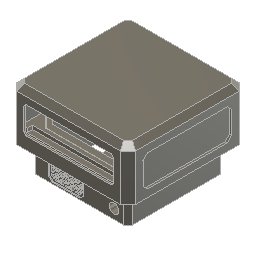
body (Autodesk Fusion 360 design; units mm, degrees)
part number: 2025-12-12-12-39-30-884
part number: 2025-12-12-12-40-35-354
part number: 2025-12-12-12-40-41-238
part number: 2025-12-13-11-33-40-663
Autodesk Fusion 360 part; units mm, degrees
(part 1 of 2)
sketch "Sketch1" plane through (0, 0, 0) normal (0, 1, 0) x (1, 0, 0) in component "Bottom"
  line L0 (-45, 45) -> (45, 45)
  line L1 (45, 45) -> (45, -45)
  line L2 (45, -45) -> (-45, -45)
  line L3 (-45, -45) -> (-45, 45)
  line L4 (-45, 45) -> (45, -45) construction
  line L5 (45, 45) -> (-45, -45) construction
  line L6 (37, -37) -> (-37, -37)
  line L7 (-37, -37) -> (-37, 37)
  line L8 (-37, 37) -> (37, 37)
  line L9 (37, 37) -> (37, -37)
  dimension "d1" = 90
  dimension "d2" = 90
  dimension "d3" = 8
  constraint horizontal L0
  constraint perpendicular L0 L1
  constraint parallel L0 L2
  constraint parallel L1 L3
  constraint coincident L4 origin
  constraint coincident L5 origin
  measures "d1" distance of L1.end L2.end
  measures "d2" distance of L0.end L1.end
extrude "Extrude1" add sketch "Sketch1" along normal blind 40 makes body 1 in component "Bottom"
sketch "Sketch2" plane through (0, 0, 0) normal (0, 0, 1) x (1, 0, 0) in component "Bottom"
ref_plane "WorkPlane1" through (0, 25, 0) normal (0, 1, 0) x (0, 0, 1) in component "Top"
sketch "Sketch1 (2)" plane through (0, 25, 0) normal (0, 1, 0) x (1, 0, 0) in component "Top"
  line L0 (55, 55) -> (-55, 55)
  line L1 (-55, 55) -> (-55, -55)
  line L2 (-55, -55) -> (55, -55)
  line L3 (55, -55) -> (55, 55)
  line L4 (55, 55) -> (-55, -55) construction
  line L5 (-55, 55) -> (55, -55) construction
  dimension "d7" = 110
  dimension "d8" = 110
  constraint horizontal L0
  constraint perpendicular L0 L1
  constraint parallel L0 L2
  constraint parallel L1 L3
  constraint coincident L4 origin
  constraint coincident L5 origin
  measures "d7" distance of L1.end L2.end
  measures "d8" distance of L0.end L1.end
extrude "Extrude1'" add sketch "Sketch1 (2)" along normal blind 48 separate body makes body 2 in component "Top"
shell "Shell1" thickness 8 removed faces 1 at (-18.3333, 25, -18.3333) on bodies 2 in component "Top"
sketch "Sketch2 (2)" plane through (0, 25, 0) normal (0, -1, 0) x (1, 0, 0) in component "Top"
  line L0 (-47, 47) -> (47, 47)
  line L1 (47, 47) -> (47, -47)
  line L2 (47, -47) -> (-47, -47)
  line L3 (-47, -47) -> (-47, 47)
  line L4 (55, -55) -> (55, 55)
  line L5 (55, 55) -> (-55, 55)
  line L6 (-55, 55) -> (-55, -55)
  line L7 (-55, -55) -> (55, -55)
  line L8 (51, -51) -> (-51, -51)
  line L9 (-51, -51) -> (-51, 51)
  line L10 (-51, 51) -> (51, 51)
  line L11 (51, 51) -> (51, -51)
  dimension "d12" = -4
extrude "Extrude2" cut sketch "Sketch2 (2)" against normal blind 10 contours L8 L9 L10 L11 bodies 2 in component "Top"
sketch "Sketch3" plane through (0, 0, 55) normal (0, 0, 1) x (1, 0, 0) in component "Top"
  line L0 (-55, 25) -> (55, 25)
  line L1 (55, 25) -> (55, 73)
  line L2 (55, 73) -> (-55, 73)
  line L3 (-55, 73) -> (-55, 25)
  line L4 (0, 73) -> (0, 25) construction
  line L5 (-41.5, 61.5) -> (41.5, 61.5)
  line L6 (41.5, 61.5) -> (41.5, 36.5)
  line L7 (41.5, 36.5) -> (-41.5, 36.5)
  line L8 (-41.5, 36.5) -> (-41.5, 61.5)
  line L9 (-41.5, 61.5) -> (41.5, 36.5) construction
  line L10 (41.5, 61.5) -> (-41.5, 36.5) construction
  line L11 (50.5, 66) -> (-50.5, 66)
  line L12 (-50.5, 66) -> (-50.5, 32)
  line L13 (-50.5, 32) -> (50.5, 32)
  line L14 (50.5, 32) -> (50.5, 66)
  line L15 (50.5, 66) -> (-50.5, 32) construction
  line L16 (-50.5, 66) -> (50.5, 32) construction
  point P0 (0, 49)
  point P1 (0, 49)
  dimension "d15" = 83
  dimension "d16" = 25
  dimension "d29" = 101
  dimension "d30" = 34
  constraint midpoint L2 L4.start
  constraint midpoint L0 L4.end
  constraint horizontal L5
  constraint perpendicular L5 L6
  constraint parallel L5 L7
  constraint parallel L6 L8
  constraint coincident L9 P1
  constraint coincident L10 P1
  constraint midpoint L4 P1
  constraint horizontal L11
  constraint perpendicular L11 L12
  constraint parallel L11 L13
  constraint parallel L12 L14
  constraint coincident L15 P1
  constraint coincident L16 P1
  constraint coincident P1 P0
  measures "d15" distance of L6.end L7.end
  measures "d16" distance of L5.end L6.end
  measures "d29" distance of L12.end L13.end
  measures "d30" distance of L11.end L12.end
extrude "Extrude3" cut sketch "Sketch3" against normal blind 8 contours L5 L6 L7 L8 bodies 2 in component "Top"
sketch "Sketch3 (2)" plane through (0, 0, 45) normal (0, 0, 1) x (1, 0, 0) in component "Bottom"
  line L0 (-45, 0) -> (45, 0)
  line L1 (45, 0) -> (45, 40)
  line L2 (45, 40) -> (-45, 40)
  line L3 (-45, 40) -> (-45, 0)
sketch "Sketch4" plane through (0, 40, 0) normal (0, 1, 0) x (-1, 0, 0) in component "Bottom"
  line L0 (37, -37) -> (-37, -37)
  line L1 (-37, -37) -> (-37, 37)
  line L2 (-37, 37) -> (37, 37)
  line L3 (37, 37) -> (37, -37)
  line L4 (45, 45) -> (-45, 45)
  line L5 (-45, 45) -> (-45, -45)
  line L6 (-45, -45) -> (45, -45)
  line L7 (45, -45) -> (45, 45)
  line L8 (43, 43) -> (-43, 43)
  line L9 (-43, 43) -> (-43, -43)
  line L10 (-43, -43) -> (43, -43)
  line L11 (43, -43) -> (43, 43)
  dimension "d20" = -2
extrude "Extrude2'" cut sketch "Sketch4" against normal blind 12 contours L4 L5 L6 L7 bodies 1 in component "Bottom"
sketch "Sketch4 (2)" plane through (0, 35, 0) normal (0, -1, 0) x (1, 0, 0) in component "Top"
  line L0 (47, -47) -> (-47, -47)
  line L1 (-47, -47) -> (-47, 47)
  line L2 (-47, 47) -> (47, 47)
  line L3 (47, 47) -> (47, -47)
  line L4 (51, 51) -> (-51, 51)
  line L5 (-51, 51) -> (-51, -51)
  line L6 (-51, -51) -> (51, -51)
  line L7 (51, -51) -> (51, 51)
  line L8 (43, -43) -> (-43, -43)
  line L9 (-43, -43) -> (-43, 43)
  line L10 (-43, 43) -> (43, 43)
  line L11 (43, 43) -> (43, -43)
  line L12 (-37, -37) -> (37, -37)
  line L13 (37, -37) -> (37, 37)
  line L14 (37, 37) -> (-37, 37)
  line L15 (-37, 37) -> (-37, -37)
extrude "Extrude4" add sketch "Sketch4 (2)" against normal blind 5 contours L0 L1 L2 L3 bodies 2 in component "Top"
sketch "Sketch5" plane through (0, 40, 0) normal (0, 1, 0) x (-1, 0, 0) in component "Top"
  line L0 (-43, 43) -> (43, 43)
  line L1 (43, 43) -> (43, -43)
  line L2 (43, -43) -> (-43, -43)
  line L3 (-43, -43) -> (-43, 43)
  line L4 (47, 47) -> (41.5, 47)
  line L5 (-47, 47) -> (-47, -47)
  line L6 (-47, -47) -> (47, -47)
  line L7 (47, -47) -> (47, 47)
  line L8 (43, -33) -> (33, -43)
  line L9 (43, -33) -> (43, -43)
  line L10 (43, -43) -> (33, -43)
  line L11 (-43, -43) -> (-33, -43)
  line L12 (-33, -43) -> (-43, -33)
  line L13 (-43, -43) -> (-43, -33)
  line L14 (-43, 43) -> (-43, 33)
  line L15 (-43, 33) -> (-33, 43)
  line L16 (-33, 43) -> (-43, 43)
  line L17 (43, 43) -> (43, 33)
  line L18 (43, 33) -> (33, 43)
  line L19 (33, 43) -> (43, 43)
  line L20 (41.5, 47) -> (-41.5, 47)
  line L21 (-41.5, 47) -> (-47, 47)
  dimension "d25" = 10
  constraint coincident L1 L8.start
  constraint coincident L2 L8.end
  constraint coincident L1.end L2.start
  constraint coincident L2.end L3.start
  constraint coincident L2 L11.end
  constraint coincident L3 L12.end
  constraint coincident L0.start L3.end
  constraint coincident L3 L14.end
  constraint coincident L0 L15.end
  constraint coincident L0.end L1.start
  constraint coincident L1 L17.end
  constraint coincident L0 L18.end
  constraint equal L9 L10
  constraint equal L10 L11
  constraint equal L11 L13
  constraint equal L17 L19
  constraint equal L10 L17
  constraint equal L14 L16
  constraint equal L10 L14
  measures "d25" distance of L8.end L1.end
extrude "Extrude5" add sketch "Sketch5" against normal blind 2 contours L0 L3 L14 L15 L16 | L0 L1 L17 L18 L19 | L2 L3 L11 L12 L13 | L1 L2 L8 L9 L10 bodies 2 in component "Top"
combine "Combine1" operation cut target body 1 tool bodies 2 keep tools in component "Bottom"
move_face "OffsetFaces1" offset -0.2 8 faces at (-43, 36, -11) (11, 36, -43) (-39.6667, 39.3333, -36.3333) (43, 36, 11) (36.3333, 39.3333, -39.6667) (-11, 36, 43) (39.6667, 39.3333, 36.3333) (-39.6667, 39.3333, 36.3333) on bodies 2 in component "Top"
extrude "Extrude6" cut 1 faces at (-45.1667, 55.5, 47) along direction (0, 0, 1) blind 6.5 on bodies 2 bodies 2 in component "Top"
sketch "Sketch6" plane through (0, 40, 0) normal (0, 1, 0) x (-1, 0, 0) in component "Top"
  line L0 (-33.0828, 43.2) -> (33.0828, 43.2)
  line L1 (33.0828, 43.2) -> (43.2, 33.0828)
  line L2 (43.2, 33.0828) -> (43.2, -33.0828)
  line L3 (43.2, -33.0828) -> (33.0828, -43.2)
  line L4 (33.0828, -43.2) -> (-33.0828, -43.2)
  line L5 (-33.0828, -43.2) -> (-43.2, -33.0828)
  line L6 (-43.2, -33.0828) -> (-43.2, 33.0828)
  line L7 (-43.2, 33.0828) -> (-33.0828, 43.2)
  line L8 (41.5, 47) -> (-41.5, 47)
  line L9 (-41.5, 47) -> (-41.5, 53.5)
  line L10 (-41.5, 53.5) -> (-47, 53.5)
  line L11 (-47, 53.5) -> (-47, -47)
  line L12 (-47, -47) -> (47, -47)
  line L13 (47, -47) -> (47, 53.5)
  line L14 (47, 53.5) -> (41.5, 53.5)
  line L15 (41.5, 53.5) -> (41.5, 47)
  line L16 (47, 53.5) -> (-47, 53.5)
  line L17 (-47, 53.5) -> (-47, 52)
  line L18 (-47, 52) -> (47, 52)
  line L19 (47, 52) -> (47, 53.5)
  dimension "d33" = 1.5
  constraint horizontal L16
  constraint vertical L17
  constraint horizontal L18
  constraint vertical L19
  constraint coincident L11 L17.end
  constraint coincident L13.end L14.start
  measures "d33" distance of L13.end L18.end
extrude "Extrude7" cut sketch "Sketch6" against normal blind 5 contours L9 L15 L16 L18 | L13 L14 L15 L16 L18 L19 | L9 L10 L11 L16 L17 L18 bodies 2 in component "Top"
chamfer "Chamfer1" distance 7 angle 45 4 edges at (-55, 49, 55) (55, 49, 55) (55, 49, -55) (-55, 49, -55) on bodies 2 in component "Top"
chamfer "Chamfer2" distance 5 angle 45 4 edges at (51, 30, 51) (-51, 30, 51) (51, 30, -51) (-51, 30, -51) on bodies 2 in component "Top"
chamfer "Chamfer3" distance 4 angle 45 2 edges at (-47, 52.5, -47) (47, 52.5, -47) on bodies 2 in component "Top"
chamfer "Chamfer4" distance 5 angle 45 8 edges at (-55, 73, 0) (-51.5, 73, 51.5) (0, 73, 55) (51.5, 73, 51.5) (55, 73, 0) (0, 73, -55) (51.5, 73, -51.5) (-51.5, 73, -51.5) on bodies 2 in component "Top"
chamfer "Chamfer1'" distance 4 angle 45 12 edges at (-45, 14, -45) (-45, 14, 45) (45, 14, -45) (-43, 33, -43) (-43, 33, 43) (45, 14, 45) (43, 33, 43) (43, 33, -43) (-37, 20, 37) (37, 20, 37) (37, 20, -37) (-37, 20, -37) on bodies 1 in component "Bottom"
sketch "Sketch5 (2)" plane through (0, 0, 37) normal (0, 0, -1) x (-1, 0, 0) in component "Bottom"
  line L0 (-33, 40) -> (-33, 0)
  line L1 (-33, 0) -> (33, 0)
  line L2 (33, 0) -> (33, 40)
  line L3 (33, 40) -> (-33, 40)
  line L4 (-2, 23) -> (27, 23)
  line L5 (27, 23) -> (27, 3)
  line L6 (27, 3) -> (-2, 3)
  line L7 (-2, 3) -> (-2, 23)
  line L8 (-2, 23) -> (27, 3) construction
  line L9 (27, 23) -> (-2, 3) construction
  line L10 (-5.5, 25.5) -> (30.5, 25.5)
  line L11 (30.5, 25.5) -> (30.5, 0.5)
  line L12 (30.5, 0.5) -> (-5.5, 0.5)
  line L13 (-5.5, 0.5) -> (-5.5, 25.5)
  line L14 (-5.5, 25.5) -> (30.5, 0.5) construction
  line L15 (30.5, 25.5) -> (-5.5, 0.5) construction
  point P0 (12.5, 13)
  point P1 (12.5, 13)
  dimension "d41" = 29
  dimension "d42" = 3
  dimension "d43" = 6
  dimension "d46" = 36
  dimension "d47" = 25
  constraint horizontal L4
  constraint perpendicular L4 L5
  constraint parallel L4 L6
  constraint parallel L5 L7
  constraint coincident L8 P1
  constraint coincident L9 P1
  constraint horizontal L10
  constraint perpendicular L10 L11
  constraint parallel L10 L12
  constraint parallel L11 L13
  constraint coincident L14 P1
  constraint coincident L15 P1
  constraint coincident P1 P0
  measures "d41" distance of L5.end L6.end
  measures "d42" distance of L1 L6
  measures "d43" distance of L2 L5
  measures "d46" distance of L11.end L12.end
  measures "d47" distance of L10.end L11.end
sketch "Sketch6 (2)" plane through (0, 0, 45) normal (0, 0, 1) x (1, 0, 0) in component "Bottom"
  line L0 (2, 23) -> (-27, 23)
  line L1 (2, 3) -> (2, 23)
  line L2 (-27, 23) -> (-27, 3)
  line L3 (-27, 3) -> (2, 3)
  line L4 (-13.6547, 15) -> (-14.8094, 13)
  line L5 (-14.8094, 13) -> (-13.6547, 11)
  line L6 (-13.6547, 11) -> (-11.3453, 11)
  line L7 (-11.3453, 11) -> (-10.1906, 13)
  line L8 (-10.1906, 13) -> (-11.3453, 15)
  line L9 (-11.3453, 15) -> (-13.6547, 15)
  line L10 (-11.3453, 15) -> (-10.0463, 15.75)
  line L11 (2.5111, 39) -> (0.2017, 39)
  line L12 (0.2017, 39) -> (-0.953, 37)
  line L13 (-0.953, 37) -> (0.2017, 35)
  line L14 (0.2017, 35) -> (2.5111, 35)
  line L15 (2.5111, 35) -> (3.6658, 37)
  line L16 (3.6658, 37) -> (2.5111, 39)
  line L17 (-2.1077, 36.3333) -> (-4.4171, 36.3333)
  line L18 (-4.4171, 36.3333) -> (-5.5718, 34.3333)
  line L19 (-5.5718, 34.3333) -> (-4.4171, 32.3333)
  line L20 (-4.4171, 32.3333) -> (-2.1077, 32.3333)
  line L21 (-2.1077, 32.3333) -> (-0.953, 34.3333)
  line L22 (-0.953, 34.3333) -> (-2.1077, 36.3333)
  line L23 (-6.7265, 33.6667) -> (-9.0359, 33.6667)
  line L24 (-9.0359, 33.6667) -> (-10.1906, 31.6667)
  line L25 (-10.1906, 31.6667) -> (-9.0359, 29.6667)
  line L26 (-9.0359, 29.6667) -> (-6.7265, 29.6667)
  line L27 (-6.7265, 29.6667) -> (-5.5718, 31.6667)
  line L28 (-5.5718, 31.6667) -> (-6.7265, 33.6667)
  line L29 (-11.3453, 31) -> (-13.6547, 31)
  line L30 (-13.6547, 31) -> (-14.8094, 29)
  line L31 (-14.8094, 29) -> (-13.6547, 27)
  line L32 (-13.6547, 27) -> (-11.3453, 27)
  line L33 (-11.3453, 27) -> (-10.1906, 29)
  line L34 (-10.1906, 29) -> (-11.3453, 31)
  line L35 (-15.9641, 28.3333) -> (-18.2735, 28.3333)
  line L36 (-18.2735, 28.3333) -> (-19.4282, 26.3333)
  line L37 (-19.4282, 26.3333) -> (-18.2735, 24.3333)
  line L38 (-18.2735, 24.3333) -> (-15.9641, 24.3333)
  line L39 (-15.9641, 24.3333) -> (-14.8094, 26.3333)
  line L40 (-14.8094, 26.3333) -> (-15.9641, 28.3333)
  line L41 (-20.5829, 25.6667) -> (-22.8923, 25.6667)
  line L42 (-22.8923, 25.6667) -> (-24.047, 23.6667)
  line L43 (-24.047, 23.6667) -> (-22.8923, 21.6667)
  line L44 (-22.8923, 21.6667) -> (-20.5829, 21.6667)
  line L45 (-20.5829, 21.6667) -> (-19.4282, 23.6667)
  line L46 (-19.4282, 23.6667) -> (-20.5829, 25.6667)
  line L47 (-25.2017, 23) -> (-27.5111, 23)
  line L48 (-27.5111, 23) -> (-28.6658, 21)
  line L49 (-28.6658, 21) -> (-27.5111, 19)
  line L50 (-27.5111, 19) -> (-25.2017, 19)
  line L51 (-25.2017, 19) -> (-24.047, 21)
  line L52 (-24.047, 21) -> (-25.2017, 23)
  line L53 (2.5111, 33.6667) -> (0.2017, 33.6667)
  line L54 (0.2017, 33.6667) -> (-0.953, 31.6667)
  line L55 (-0.953, 31.6667) -> (0.2017, 29.6667)
  line L56 (0.2017, 29.6667) -> (2.5111, 29.6667)
  line L57 (2.5111, 29.6667) -> (3.6658, 31.6667)
  line L58 (3.6658, 31.6667) -> (2.5111, 33.6667)
  line L59 (-2.1077, 31) -> (-4.4171, 31)
  line L60 (-4.4171, 31) -> (-5.5718, 29)
  line L61 (-5.5718, 29) -> (-4.4171, 27)
  line L62 (-4.4171, 27) -> (-2.1077, 27)
  line L63 (-2.1077, 27) -> (-0.953, 29)
  line L64 (-0.953, 29) -> (-2.1077, 31)
  line L65 (-6.7265, 28.3333) -> (-9.0359, 28.3333)
  line L66 (-9.0359, 28.3333) -> (-10.1906, 26.3333)
  line L67 (-10.1906, 26.3333) -> (-9.0359, 24.3333)
  line L68 (-9.0359, 24.3333) -> (-6.7265, 24.3333)
  line L69 (-6.7265, 24.3333) -> (-5.5718, 26.3333)
  line L70 (-5.5718, 26.3333) -> (-6.7265, 28.3333)
  line L71 (-11.3453, 25.6667) -> (-13.6547, 25.6667)
  line L72 (-13.6547, 25.6667) -> (-14.8094, 23.6667)
  line L73 (-14.8094, 23.6667) -> (-13.6547, 21.6667)
  line L74 (-13.6547, 21.6667) -> (-11.3453, 21.6667)
  line L75 (-11.3453, 21.6667) -> (-10.1906, 23.6667)
  line L76 (-10.1906, 23.6667) -> (-11.3453, 25.6667)
  line L77 (-15.9641, 23) -> (-18.2735, 23)
  line L78 (-18.2735, 23) -> (-19.4282, 21)
  line L79 (-19.4282, 21) -> (-18.2735, 19)
  line L80 (-18.2735, 19) -> (-15.9641, 19)
  line L81 (-15.9641, 19) -> (-14.8094, 21)
  line L82 (-14.8094, 21) -> (-15.9641, 23)
  line L83 (-20.5829, 20.3333) -> (-22.8923, 20.3333)
  line L84 (-22.8923, 20.3333) -> (-24.047, 18.3333)
  line L85 (-24.047, 18.3333) -> (-22.8923, 16.3333)
  line L86 (-22.8923, 16.3333) -> (-20.5829, 16.3333)
  line L87 (-20.5829, 16.3333) -> (-19.4282, 18.3333)
  line L88 (-19.4282, 18.3333) -> (-20.5829, 20.3333)
  line L89 (-25.2017, 17.6667) -> (-27.5111, 17.6667)
  line L90 (-27.5111, 17.6667) -> (-28.6658, 15.6667)
  line L91 (-28.6658, 15.6667) -> (-27.5111, 13.6667)
  line L92 (-27.5111, 13.6667) -> (-25.2017, 13.6667)
  line L93 (-25.2017, 13.6667) -> (-24.047, 15.6667)
  line L94 (-24.047, 15.6667) -> (-25.2017, 17.6667)
  line L95 (2.5111, 28.3333) -> (0.2017, 28.3333)
  line L96 (0.2017, 28.3333) -> (-0.953, 26.3333)
  line L97 (-0.953, 26.3333) -> (0.2017, 24.3333)
  line L98 (0.2017, 24.3333) -> (2.5111, 24.3333)
  line L99 (2.5111, 24.3333) -> (3.6658, 26.3333)
  line L100 (3.6658, 26.3333) -> (2.5111, 28.3333)
  line L101 (-2.1077, 25.6667) -> (-4.4171, 25.6667)
  line L102 (-4.4171, 25.6667) -> (-5.5718, 23.6667)
  line L103 (-5.5718, 23.6667) -> (-4.4171, 21.6667)
  line L104 (-4.4171, 21.6667) -> (-2.1077, 21.6667)
  line L105 (-2.1077, 21.6667) -> (-0.953, 23.6667)
  line L106 (-0.953, 23.6667) -> (-2.1077, 25.6667)
  line L107 (-6.7265, 23) -> (-9.0359, 23)
  line L108 (-9.0359, 23) -> (-10.1906, 21)
  line L109 (-10.1906, 21) -> (-9.0359, 19)
  line L110 (-9.0359, 19) -> (-6.7265, 19)
  line L111 (-6.7265, 19) -> (-5.5718, 21)
  line L112 (-5.5718, 21) -> (-6.7265, 23)
  line L113 (-11.3453, 20.3333) -> (-13.6547, 20.3333)
  line L114 (-13.6547, 20.3333) -> (-14.8094, 18.3333)
  line L115 (-14.8094, 18.3333) -> (-13.6547, 16.3333)
  line L116 (-13.6547, 16.3333) -> (-11.3453, 16.3333)
  line L117 (-11.3453, 16.3333) -> (-10.1906, 18.3333)
  line L118 (-10.1906, 18.3333) -> (-11.3453, 20.3333)
  line L119 (-15.9641, 17.6667) -> (-18.2735, 17.6667)
  line L120 (-18.2735, 17.6667) -> (-19.4282, 15.6667)
  line L121 (-19.4282, 15.6667) -> (-18.2735, 13.6667)
  line L122 (-18.2735, 13.6667) -> (-15.9641, 13.6667)
  line L123 (-15.9641, 13.6667) -> (-14.8094, 15.6667)
  line L124 (-14.8094, 15.6667) -> (-15.9641, 17.6667)
  line L125 (-20.5829, 15) -> (-22.8923, 15)
  line L126 (-22.8923, 15) -> (-24.047, 13)
  line L127 (-24.047, 13) -> (-22.8923, 11)
  line L128 (-22.8923, 11) -> (-20.5829, 11)
  line L129 (-20.5829, 11) -> (-19.4282, 13)
  line L130 (-19.4282, 13) -> (-20.5829, 15)
  line L131 (-25.2017, 12.3333) -> (-27.5111, 12.3333)
  line L132 (-27.5111, 12.3333) -> (-28.6658, 10.3333)
  line L133 (-28.6658, 10.3333) -> (-27.5111, 8.3333)
  line L134 (-27.5111, 8.3333) -> (-25.2017, 8.3333)
  line L135 (-25.2017, 8.3333) -> (-24.047, 10.3333)
  line L136 (-24.047, 10.3333) -> (-25.2017, 12.3333)
  line L137 (2.5111, 23) -> (0.2017, 23)
  line L138 (0.2017, 23) -> (-0.953, 21)
  line L139 (-0.953, 21) -> (0.2017, 19)
  line L140 (0.2017, 19) -> (2.5111, 19)
  line L141 (2.5111, 19) -> (3.6658, 21)
  line L142 (3.6658, 21) -> (2.5111, 23)
  line L143 (-2.1077, 20.3333) -> (-4.4171, 20.3333)
  line L144 (-4.4171, 20.3333) -> (-5.5718, 18.3333)
  line L145 (-5.5718, 18.3333) -> (-4.4171, 16.3333)
  line L146 (-4.4171, 16.3333) -> (-2.1077, 16.3333)
  line L147 (-2.1077, 16.3333) -> (-0.953, 18.3333)
  line L148 (-0.953, 18.3333) -> (-2.1077, 20.3333)
  line L149 (-6.7265, 17.6667) -> (-9.0359, 17.6667)
  line L150 (-9.0359, 17.6667) -> (-10.1906, 15.6667)
  line L151 (-10.1906, 15.6667) -> (-9.0359, 13.6667)
  line L152 (-9.0359, 13.6667) -> (-6.7265, 13.6667)
  line L153 (-6.7265, 13.6667) -> (-5.5718, 15.6667)
  line L154 (-5.5718, 15.6667) -> (-6.7265, 17.6667)
  line L155 (-15.9641, 12.3333) -> (-18.2735, 12.3333)
  line L156 (-18.2735, 12.3333) -> (-19.4282, 10.3333)
  line L157 (-19.4282, 10.3333) -> (-18.2735, 8.3333)
  line L158 (-18.2735, 8.3333) -> (-15.9641, 8.3333)
  line L159 (-15.9641, 8.3333) -> (-14.8094, 10.3333)
  line L160 (-14.8094, 10.3333) -> (-15.9641, 12.3333)
  line L161 (-20.5829, 9.6667) -> (-22.8923, 9.6667)
  line L162 (-22.8923, 9.6667) -> (-24.047, 7.6667)
  line L163 (-24.047, 7.6667) -> (-22.8923, 5.6667)
  line L164 (-22.8923, 5.6667) -> (-20.5829, 5.6667)
  line L165 (-20.5829, 5.6667) -> (-19.4282, 7.6667)
  line L166 (-19.4282, 7.6667) -> (-20.5829, 9.6667)
  line L167 (-25.2017, 7) -> (-27.5111, 7)
  line L168 (-27.5111, 7) -> (-28.6658, 5)
  line L169 (-28.6658, 5) -> (-27.5111, 3)
  line L170 (-27.5111, 3) -> (-25.2017, 3)
  line L171 (-25.2017, 3) -> (-24.047, 5)
  line L172 (-24.047, 5) -> (-25.2017, 7)
  line L173 (2.5111, 17.6667) -> (0.2017, 17.6667)
  line L174 (0.2017, 17.6667) -> (-0.953, 15.6667)
  line L175 (-0.953, 15.6667) -> (0.2017, 13.6667)
  line L176 (0.2017, 13.6667) -> (2.5111, 13.6667)
  line L177 (2.5111, 13.6667) -> (3.6658, 15.6667)
  line L178 (3.6658, 15.6667) -> (2.5111, 17.6667)
  line L179 (-2.1077, 15) -> (-4.4171, 15)
  line L180 (-4.4171, 15) -> (-5.5718, 13)
  line L181 (-5.5718, 13) -> (-4.4171, 11)
  line L182 (-4.4171, 11) -> (-2.1077, 11)
  line L183 (-2.1077, 11) -> (-0.953, 13)
  line L184 (-0.953, 13) -> (-2.1077, 15)
  line L185 (-6.7265, 12.3333) -> (-9.0359, 12.3333)
  line L186 (-9.0359, 12.3333) -> (-10.1906, 10.3333)
  line L187 (-10.1906, 10.3333) -> (-9.0359, 8.3333)
  line L188 (-9.0359, 8.3333) -> (-6.7265, 8.3333)
  line L189 (-6.7265, 8.3333) -> (-5.5718, 10.3333)
  line L190 (-5.5718, 10.3333) -> (-6.7265, 12.3333)
  line L191 (-11.3453, 9.6667) -> (-13.6547, 9.6667)
  line L192 (-13.6547, 9.6667) -> (-14.8094, 7.6667)
  line L193 (-14.8094, 7.6667) -> (-13.6547, 5.6667)
  line L194 (-13.6547, 5.6667) -> (-11.3453, 5.6667)
  line L195 (-11.3453, 5.6667) -> (-10.1906, 7.6667)
  line L196 (-10.1906, 7.6667) -> (-11.3453, 9.6667)
  line L197 (-15.9641, 7) -> (-18.2735, 7)
  line L198 (-18.2735, 7) -> (-19.4282, 5)
  line L199 (-19.4282, 5) -> (-18.2735, 3)
  line L200 (-18.2735, 3) -> (-15.9641, 3)
  line L201 (-15.9641, 3) -> (-14.8094, 5)
  line L202 (-14.8094, 5) -> (-15.9641, 7)
  line L203 (-20.5829, 4.3333) -> (-22.8923, 4.3333)
  line L204 (-22.8923, 4.3333) -> (-24.047, 2.3333)
  line L205 (-24.047, 2.3333) -> (-22.8923, 0.3333)
  line L206 (-22.8923, 0.3333) -> (-20.5829, 0.3333)
  line L207 (-20.5829, 0.3333) -> (-19.4282, 2.3333)
  line L208 (-19.4282, 2.3333) -> (-20.5829, 4.3333)
  line L209 (-25.2017, 1.6667) -> (-27.5111, 1.6667)
  line L210 (-27.5111, 1.6667) -> (-28.6658, -0.3333)
  line L211 (-28.6658, -0.3333) -> (-27.5111, -2.3333)
  line L212 (-27.5111, -2.3333) -> (-25.2017, -2.3333)
  line L213 (-25.2017, -2.3333) -> (-24.047, -0.3333)
  line L214 (-24.047, -0.3333) -> (-25.2017, 1.6667)
  line L215 (2.5111, 12.3333) -> (0.2017, 12.3333)
  line L216 (0.2017, 12.3333) -> (-0.953, 10.3333)
  line L217 (-0.953, 10.3333) -> (0.2017, 8.3333)
  line L218 (0.2017, 8.3333) -> (2.5111, 8.3333)
  line L219 (2.5111, 8.3333) -> (3.6658, 10.3333)
  line L220 (3.6658, 10.3333) -> (2.5111, 12.3333)
  line L221 (-2.1077, 9.6667) -> (-4.4171, 9.6667)
  line L222 (-4.4171, 9.6667) -> (-5.5718, 7.6667)
  line L223 (-5.5718, 7.6667) -> (-4.4171, 5.6667)
  line L224 (-4.4171, 5.6667) -> (-2.1077, 5.6667)
  line L225 (-2.1077, 5.6667) -> (-0.953, 7.6667)
  line L226 (-0.953, 7.6667) -> (-2.1077, 9.6667)
  line L227 (-6.7265, 7) -> (-9.0359, 7)
  line L228 (-9.0359, 7) -> (-10.1906, 5)
  line L229 (-10.1906, 5) -> (-9.0359, 3)
  line L230 (-9.0359, 3) -> (-6.7265, 3)
  line L231 (-6.7265, 3) -> (-5.5718, 5)
  line L232 (-5.5718, 5) -> (-6.7265, 7)
  line L233 (-11.3453, 4.3333) -> (-13.6547, 4.3333)
  line L234 (-13.6547, 4.3333) -> (-14.8094, 2.3333)
  line L235 (-14.8094, 2.3333) -> (-13.6547, 0.3333)
  line L236 (-13.6547, 0.3333) -> (-11.3453, 0.3333)
  line L237 (-11.3453, 0.3333) -> (-10.1906, 2.3333)
  line L238 (-10.1906, 2.3333) -> (-11.3453, 4.3333)
  line L239 (-15.9641, 1.6667) -> (-18.2735, 1.6667)
  line L240 (-18.2735, 1.6667) -> (-19.4282, -0.3333)
  line L241 (-19.4282, -0.3333) -> (-18.2735, -2.3333)
  line L242 (-18.2735, -2.3333) -> (-15.9641, -2.3333)
  line L243 (-15.9641, -2.3333) -> (-14.8094, -0.3333)
  line L244 (-14.8094, -0.3333) -> (-15.9641, 1.6667)
  line L245 (-20.5829, -1) -> (-22.8923, -1)
  line L246 (-22.8923, -1) -> (-24.047, -3)
  line L247 (-24.047, -3) -> (-22.8923, -5)
  line L248 (-22.8923, -5) -> (-20.5829, -5)
  line L249 (-20.5829, -5) -> (-19.4282, -3)
  line L250 (-19.4282, -3) -> (-20.5829, -1)
  line L251 (-25.2017, -3.6667) -> (-27.5111, -3.6667)
  line L252 (-27.5111, -3.6667) -> (-28.6658, -5.6667)
  line L253 (-28.6658, -5.6667) -> (-27.5111, -7.6667)
  line L254 (-27.5111, -7.6667) -> (-25.2017, -7.6667)
  line L255 (-25.2017, -7.6667) -> (-24.047, -5.6667)
  line L256 (-24.047, -5.6667) -> (-25.2017, -3.6667)
  line L257 (2.5111, 7) -> (0.2017, 7)
  line L258 (0.2017, 7) -> (-0.953, 5)
  line L259 (-0.953, 5) -> (0.2017, 3)
  line L260 (0.2017, 3) -> (2.5111, 3)
  line L261 (2.5111, 3) -> (3.6658, 5)
  line L262 (3.6658, 5) -> (2.5111, 7)
  line L263 (-2.1077, 4.3333) -> (-4.4171, 4.3333)
  line L264 (-4.4171, 4.3333) -> (-5.5718, 2.3333)
  line L265 (-5.5718, 2.3333) -> (-4.4171, 0.3333)
  line L266 (-4.4171, 0.3333) -> (-2.1077, 0.3333)
  line L267 (-2.1077, 0.3333) -> (-0.953, 2.3333)
  line L268 (-0.953, 2.3333) -> (-2.1077, 4.3333)
  line L269 (-6.7265, 1.6667) -> (-9.0359, 1.6667)
  line L270 (-9.0359, 1.6667) -> (-10.1906, -0.3333)
  line L271 (-10.1906, -0.3333) -> (-9.0359, -2.3333)
  line L272 (-9.0359, -2.3333) -> (-6.7265, -2.3333)
  line L273 (-6.7265, -2.3333) -> (-5.5718, -0.3333)
  line L274 (-5.5718, -0.3333) -> (-6.7265, 1.6667)
  line L275 (-11.3453, -1) -> (-13.6547, -1)
  line L276 (-13.6547, -1) -> (-14.8094, -3)
  line L277 (-14.8094, -3) -> (-13.6547, -5)
  line L278 (-13.6547, -5) -> (-11.3453, -5)
  line L279 (-11.3453, -5) -> (-10.1906, -3)
  line L280 (-10.1906, -3) -> (-11.3453, -1)
  line L281 (-15.9641, -3.6667) -> (-18.2735, -3.6667)
  line L282 (-18.2735, -3.6667) -> (-19.4282, -5.6667)
  line L283 (-19.4282, -5.6667) -> (-18.2735, -7.6667)
  line L284 (-18.2735, -7.6667) -> (-15.9641, -7.6667)
  line L285 (-15.9641, -7.6667) -> (-14.8094, -5.6667)
  line L286 (-14.8094, -5.6667) -> (-15.9641, -3.6667)
  line L287 (-20.5829, -6.3333) -> (-22.8923, -6.3333)
  line L288 (-22.8923, -6.3333) -> (-24.047, -8.3333)
  line L289 (-24.047, -8.3333) -> (-22.8923, -10.3333)
  line L290 (-22.8923, -10.3333) -> (-20.5829, -10.3333)
  line L291 (-20.5829, -10.3333) -> (-19.4282, -8.3333)
  line L292 (-19.4282, -8.3333) -> (-20.5829, -6.3333)
  line L293 (-25.2017, -9) -> (-27.5111, -9)
  line L294 (-27.5111, -9) -> (-28.6658, -11)
  line L295 (-28.6658, -11) -> (-27.5111, -13)
  line L296 (-27.5111, -13) -> (-25.2017, -13)
  line L297 (-25.2017, -13) -> (-24.047, -11)
  line L298 (-24.047, -11) -> (-25.2017, -9)
  point P0 (-12.5, 13)
  point P1 (-12.5, 13)
  dimension "d51" = 2
  dimension "d52" = 1.5
  dimension "d55" = 16
  dimension "d56" = 16
  constraint coincident P1 P0
  constraint perpendicular L8 L10
  measures "d51" distance of P1 L9
  measures "d52" distance of L8.end L10.end
extrude "Extrude5'" cut sketch "Sketch5 (2)" against normal blind 6 contours L4 L5 L6 L7 bodies 1 in component "Bottom"
extrude "Extrude6'" cut sketch "Sketch5 (2)" against normal blind 4 contours L10 L11 L12 L13 bodies 1 in component "Bottom"
extrude "Extrude7'" cut sketch "Sketch6 (2)" against normal blind 2 contours L0 L1 L137 L138 L139 L140 | L0 L103 L104 L105 | L1 L173 L174 L175 L176 | L0 L107 L108 L109 L110 L111 L112 | L1 L215 L216 L217 L218 | L0 L73 L74 L75 | L1 L3 L257 L258 L259 L260 | L0 L77 L78 L79 L80 L81 L82 | L3 L263 L264 L268 | L0 L43 L44 L45 | L3 L227 L228 L229 L230 L231 L232 | L0 L2 L47 L50 L51 L52 | L3 L233 L234 L238 | L2 L89 L92 L93 L94 | L3 L197 L198 L199 L200 L201 L202 | L2 L131 L134 L135 L136 | L3 L203 L204 L208 | L2 L3 L167 L170 L171 L172 | L4 L5 L6 L7 L8 L9 | L83 L84 L85 L86 L87 L88 | L113 L114 L115 L116 L117 L118 | L119 L120 L121 L122 L123 L124 | L125 L126 L127 L128 L129 L130 | L143 L144 L145 L146 L147 L148 | L149 L150 L151 L152 L153 L154 | L155 L156 L157 L158 L159 L160 | L161 L162 L163 L164 L165 L166 | L179 L180 L181 L182 L183 L184 | L185 L186 L187 L188 L189 L190 | L191 L192 L193 L194 L195 L196 | L221 L222 L223 L224 L225 L226 bodies 1 in component "Bottom"
chamfer "Chamfer3'" distance 3 angle 45 8 edges at (-27, 23, 43) (-27, 3, 43) (2, 3, 43) (2, 23, 43) (-30.5, 25.5, 39) (-30.5, 0.5, 39) (5.5, 0.5, 39) (5.5, 25.5, 39) on bodies 1 in component "Bottom"
sketch "Sketch7" plane through (0, 0, 45) normal (0, 0, 1) x (1, 0, 0) in component "Bottom"
  line L0 (-5.1869, 23) -> (-1.3379, 23)
  line L1 (-1.3379, 23) -> (-2.1077, 21.6667)
  line L2 (-2.1077, 21.6667) -> (-4.4171, 21.6667)
  line L3 (-4.4171, 21.6667) -> (-5.1869, 23)
  line L4 (-4.4171, 15) -> (-2.1077, 15)
  line L5 (-2.1077, 15) -> (-0.953, 13)
  line L6 (-0.953, 13) -> (-2.1077, 11)
  line L7 (-2.1077, 11) -> (-4.4171, 11)
  line L8 (-4.4171, 11) -> (-5.5718, 13)
  line L9 (-5.5718, 13) -> (-4.4171, 15)
  line L10 (-9.0359, 12.3333) -> (-6.7265, 12.3333)
  line L11 (-6.7265, 12.3333) -> (-5.5718, 10.3333)
  line L12 (-5.5718, 10.3333) -> (-6.7265, 8.3333)
  line L13 (-6.7265, 8.3333) -> (-9.0359, 8.3333)
  line L14 (-9.0359, 8.3333) -> (-10.1906, 10.3333)
  line L15 (-10.1906, 10.3333) -> (-9.0359, 12.3333)
  line L16 (-13.6547, 20.3333) -> (-11.3453, 20.3333)
  line L17 (-11.3453, 20.3333) -> (-10.1906, 18.3333)
  line L18 (-10.1906, 18.3333) -> (-11.3453, 16.3333)
  line L19 (-11.3453, 16.3333) -> (-13.6547, 16.3333)
  line L20 (-13.6547, 16.3333) -> (-14.8094, 18.3333)
  line L21 (-14.8094, 18.3333) -> (-13.6547, 20.3333)
  line L22 (-18.2735, 7) -> (-15.9641, 7)
  line L23 (-15.9641, 7) -> (-14.8094, 5)
  line L24 (-14.8094, 5) -> (-15.9641, 3)
  line L25 (-15.9641, 3) -> (-18.2735, 3)
  line L26 (-18.2735, 3) -> (-19.4282, 5)
  line L27 (-19.4282, 5) -> (-18.2735, 7)
  line L28 (-23.6621, 23) -> (-19.8131, 23)
  line L29 (-19.8131, 23) -> (-20.5829, 21.6667)
  line L30 (-20.5829, 21.6667) -> (-22.8923, 21.6667)
  line L31 (-22.8923, 21.6667) -> (-23.6621, 23)
  line L32 (-20.5829, 4.3333) -> (-19.8131, 3)
  line L33 (-19.8131, 3) -> (-23.6621, 3)
  line L34 (-23.6621, 3) -> (-22.8923, 4.3333)
  line L35 (-22.8923, 4.3333) -> (-20.5829, 4.3333)
  line L36 (-24.7619, 22.2381) -> (-24.047, 21)
  line L37 (-24.047, 21) -> (-25.2017, 19)
  line L38 (-25.2017, 19) -> (-27, 19)
  line L39 (-27, 19) -> (-27, 20)
  line L40 (-27, 20) -> (-24.7619, 22.2381)
  line L41 (-27, 7) -> (-25.2017, 7)
  line L42 (-25.2017, 7) -> (-24.047, 5)
  line L43 (-24.047, 5) -> (-24.7619, 3.7619)
  line L44 (-24.7619, 3.7619) -> (-27, 6)
  line L45 (-27, 6) -> (-27, 7)
  line L46 (-22.8923, 20.3333) -> (-20.5829, 20.3333)
  line L47 (-20.5829, 20.3333) -> (-19.4282, 18.3333)
  line L48 (-19.4282, 18.3333) -> (-20.5829, 16.3333)
  line L49 (-20.5829, 16.3333) -> (-22.8923, 16.3333)
  line L50 (-22.8923, 16.3333) -> (-24.047, 18.3333)
  line L51 (-24.047, 18.3333) -> (-22.8923, 20.3333)
  line L52 (-18.2735, 12.3333) -> (-15.9641, 12.3333)
  line L53 (-15.9641, 12.3333) -> (-14.8094, 10.3333)
  line L54 (-14.8094, 10.3333) -> (-15.9641, 8.3333)
  line L55 (-15.9641, 8.3333) -> (-18.2735, 8.3333)
  line L56 (-18.2735, 8.3333) -> (-19.4282, 10.3333)
  line L57 (-19.4282, 10.3333) -> (-18.2735, 12.3333)
  line L58 (-14.8094, 13) -> (-13.6547, 15)
  line L59 (-13.6547, 15) -> (-11.3453, 15)
  line L60 (-11.3453, 15) -> (-10.1906, 13)
  line L61 (-10.1906, 13) -> (-11.3453, 11)
  line L62 (-11.3453, 11) -> (-13.6547, 11)
  line L63 (-13.6547, 11) -> (-14.8094, 13)
  line L64 (-9.0359, 17.6667) -> (-6.7265, 17.6667)
  line L65 (-6.7265, 17.6667) -> (-5.5718, 15.6667)
  line L66 (-5.5718, 15.6667) -> (-6.7265, 13.6667)
  line L67 (-6.7265, 13.6667) -> (-9.0359, 13.6667)
  line L68 (-9.0359, 13.6667) -> (-10.1906, 15.6667)
  line L69 (-10.1906, 15.6667) -> (-9.0359, 17.6667)
  line L70 (-4.4171, 9.6667) -> (-2.1077, 9.6667)
  line L71 (-2.1077, 9.6667) -> (-0.953, 7.6667)
  line L72 (-0.953, 7.6667) -> (-2.1077, 5.6667)
  line L73 (-2.1077, 5.6667) -> (-4.4171, 5.6667)
  line L74 (-4.4171, 5.6667) -> (-5.5718, 7.6667)
  line L75 (-5.5718, 7.6667) -> (-4.4171, 9.6667)
  line L76 (-4.4171, 20.3333) -> (-2.1077, 20.3333)
  line L77 (-2.1077, 20.3333) -> (-0.953, 18.3333)
  line L78 (-0.953, 18.3333) -> (-2.1077, 16.3333)
  line L79 (-2.1077, 16.3333) -> (-4.4171, 16.3333)
  line L80 (-4.4171, 16.3333) -> (-5.5718, 18.3333)
  line L81 (-5.5718, 18.3333) -> (-4.4171, 20.3333)
  line L82 (2, 12.3333) -> (2, 8.3333)
  line L83 (2, 8.3333) -> (0.2017, 8.3333)
  line L84 (0.2017, 8.3333) -> (-0.953, 10.3333)
  line L85 (-0.953, 10.3333) -> (0.2017, 12.3333)
  line L86 (0.2017, 12.3333) -> (2, 12.3333)
  line L87 (2, 17.6667) -> (2, 13.6667)
  line L88 (2, 13.6667) -> (0.2017, 13.6667)
  line L89 (0.2017, 13.6667) -> (-0.953, 15.6667)
  line L90 (-0.953, 15.6667) -> (0.2017, 17.6667)
  line L91 (0.2017, 17.6667) -> (2, 17.6667)
  line L92 (-9.0359, 7) -> (-6.7265, 7)
  line L93 (-6.7265, 7) -> (-5.5718, 5)
  line L94 (-5.5718, 5) -> (-6.7265, 3)
  line L95 (-6.7265, 3) -> (-9.0359, 3)
  line L96 (-9.0359, 3) -> (-10.1906, 5)
  line L97 (-10.1906, 5) -> (-9.0359, 7)
  line L98 (-14.4245, 23) -> (-10.5755, 23)
  line L99 (-10.5755, 23) -> (-11.3453, 21.6667)
  line L100 (-11.3453, 21.6667) -> (-13.6547, 21.6667)
  line L101 (-13.6547, 21.6667) -> (-14.4245, 23)
  line L102 (-11.3453, 4.3333) -> (-10.5755, 3)
  line L103 (-10.5755, 3) -> (-14.4245, 3)
  line L104 (-14.4245, 3) -> (-13.6547, 4.3333)
  line L105 (-13.6547, 4.3333) -> (-11.3453, 4.3333)
  line L106 (-18.2735, 23) -> (-15.9641, 23)
  line L107 (-15.9641, 23) -> (-14.8094, 21)
  line L108 (-14.8094, 21) -> (-15.9641, 19)
  line L109 (-15.9641, 19) -> (-18.2735, 19)
  line L110 (-18.2735, 19) -> (-19.4282, 21)
  line L111 (-19.4282, 21) -> (-18.2735, 23)
  line L112 (-22.8923, 9.6667) -> (-20.5829, 9.6667)
  line L113 (-20.5829, 9.6667) -> (-19.4282, 7.6667)
  line L114 (-19.4282, 7.6667) -> (-20.5829, 5.6667)
  line L115 (-20.5829, 5.6667) -> (-22.8923, 5.6667)
  line L116 (-22.8923, 5.6667) -> (-24.047, 7.6667)
  line L117 (-24.047, 7.6667) -> (-22.8923, 9.6667)
  line L118 (-27, 17.6667) -> (-25.2017, 17.6667)
  line L119 (-25.2017, 17.6667) -> (-24.047, 15.6667)
  line L120 (-24.047, 15.6667) -> (-25.2017, 13.6667)
  line L121 (-25.2017, 13.6667) -> (-27, 13.6667)
  line L122 (-27, 13.6667) -> (-27, 17.6667)
  line L123 (-27, 12.3333) -> (-25.2017, 12.3333)
  line L124 (-25.2017, 12.3333) -> (-24.047, 10.3333)
  line L125 (-24.047, 10.3333) -> (-25.2017, 8.3333)
  line L126 (-25.2017, 8.3333) -> (-27, 8.3333)
  line L127 (-27, 8.3333) -> (-27, 12.3333)
  line L128 (-22.8923, 15) -> (-20.5829, 15)
  line L129 (-20.5829, 15) -> (-19.4282, 13)
  line L130 (-19.4282, 13) -> (-20.5829, 11)
  line L131 (-20.5829, 11) -> (-22.8923, 11)
  line L132 (-22.8923, 11) -> (-24.047, 13)
  line L133 (-24.047, 13) -> (-22.8923, 15)
  line L134 (-18.2735, 17.6667) -> (-15.9641, 17.6667)
  line L135 (-15.9641, 17.6667) -> (-14.8094, 15.6667)
  line L136 (-14.8094, 15.6667) -> (-15.9641, 13.6667)
  line L137 (-15.9641, 13.6667) -> (-18.2735, 13.6667)
  line L138 (-18.2735, 13.6667) -> (-19.4282, 15.6667)
  line L139 (-19.4282, 15.6667) -> (-18.2735, 17.6667)
  line L140 (-13.6547, 9.6667) -> (-11.3453, 9.6667)
  line L141 (-11.3453, 9.6667) -> (-10.1906, 7.6667)
  line L142 (-10.1906, 7.6667) -> (-11.3453, 5.6667)
  line L143 (-11.3453, 5.6667) -> (-13.6547, 5.6667)
  line L144 (-13.6547, 5.6667) -> (-14.8094, 7.6667)
  line L145 (-14.8094, 7.6667) -> (-13.6547, 9.6667)
  line L146 (-9.0359, 23) -> (-6.7265, 23)
  line L147 (-6.7265, 23) -> (-5.5718, 21)
  line L148 (-5.5718, 21) -> (-6.7265, 19)
  line L149 (-6.7265, 19) -> (-9.0359, 19)
  line L150 (-9.0359, 19) -> (-10.1906, 21)
  line L151 (-10.1906, 21) -> (-9.0359, 23)
  line L152 (-2.1077, 4.3333) -> (-1.3379, 3)
  line L153 (-1.3379, 3) -> (-5.1869, 3)
  line L154 (-5.1869, 3) -> (-4.4171, 4.3333)
  line L155 (-4.4171, 4.3333) -> (-2.1077, 4.3333)
  line L156 (2, 20) -> (2, 19)
  line L157 (2, 19) -> (0.2017, 19)
  line L158 (0.2017, 19) -> (-0.953, 21)
  line L159 (-0.953, 21) -> (-0.2381, 22.2381)
  line L160 (-0.2381, 22.2381) -> (2, 20)
  line L161 (2, 7) -> (2, 6)
  line L162 (2, 6) -> (-0.2381, 3.7619)
  line L163 (-0.2381, 3.7619) -> (-0.953, 5)
  line L164 (-0.953, 5) -> (0.2017, 7)
  line L165 (0.2017, 7) -> (2, 7)
  line L166 (41, 0) -> (41, 28)
  line L167 (41, 28) -> (-41, 28)
  line L168 (-41, 28) -> (-41, 0)
  line L169 (-41, 0) -> (41, 0)
  circle A0 centre (32, 9) radius 4.5
  dimension "d64" = 9
  dimension "d65" = 9
  dimension "d66" = 9
  measures "d64" diameter of A0
  measures "d65" distance of L169 A0.centre
  measures "d66" distance of L166 A0.centre
extrude "Extrude8" cut sketch "Sketch7" against normal blind 16 contours A0 bodies 1 in component "Bottom"
sketch "Sketch7 (2)" plane through (55, 0, 0) normal (1, 0, 0) x (0, 0, -1) in component "Top"
  line L0 (48, 68) -> (-48, 68)
  line L1 (-48, 68) -> (-48, 25)
  line L2 (-48, 25) -> (48, 25)
  line L3 (48, 25) -> (48, 68)
  line L4 (-41, 32) -> (41, 32)
  line L5 (41, 32) -> (41, 61)
  line L6 (41, 61) -> (-41, 61)
  line L7 (-41, 61) -> (-41, 32)
  dimension "d69" = -7
extrude "Extrude8'" cut sketch "Sketch7 (2)" against normal blind 2 contours L4 L5 L6 L7 bodies 2 in component "Top"
chamfer "Chamfer5" distance 4 angle 45 4 edges at (54, 61, -41) (54, 32, -41) (54, 61, 41) (54, 32, 41) on bodies 2 in component "Top"
mirror "Mirror2" about plane through (0, 0, 0) normal (1, 0, 0) of "Extrude8'", "Chamfer5" in component "Top"
chamfer "Chamfer6" distance 2 angle 45 4 edges at (-41.5, 61.5, 54.25) (-41.5, 36.5, 54.25) (41.5, 36.5, 54.25) (41.5, 61.5, 54.25) on bodies 2 in component "Top"
ref_plane "WorkPlane2" through (0, 46.5, 0) normal (0.707107, 0, 0.707107) x (0.707107, 0, -0.707107) in component "Top"
mirror "Mirror3" about plane through (0, 46.5, 0) normal (0.707107, 0, 0.707107) of "Extrude8'", "Chamfer5" in component "Top"
sketch "Sketch9" plane through (0, 0, 0) normal (0, -1, 0) x (1, 0, 0) in component "Bottom"
  line L0 (45, 41) -> (41, 45)
  line L1 (41, 45) -> (-41, 45)
  line L2 (-41, 45) -> (-45, 41)
  line L3 (-45, 41) -> (-45, -41)
  line L4 (-45, -41) -> (-41, -45)
  line L5 (-41, -45) -> (41, -45)
  line L6 (41, -45) -> (45, -41)
  line L7 (45, -41) -> (45, 41)
  line L8 (-33, -37) -> (-37, -33)
  line L9 (-37, -33) -> (-37, 33)
  line L10 (-37, 33) -> (-33, 37)
  line L11 (-33, 37) -> (33, 37)
  line L12 (33, 37) -> (37, 33)
  line L13 (37, 33) -> (37, -33)
  line L14 (37, -33) -> (33, -37)
  line L15 (33, -37) -> (-33, -37)
  line L16 (-20, 45) -> (20, 45)
  line L17 (20, 45) -> (20, -45)
  line L18 (20, -45) -> (-20, -45)
  line L19 (-20, -45) -> (-20, 45)
  line L20 (-45, 45) -> (45, 45)
  line L21 (-6, 45) -> (-6, -45)
  line L22 (6, 45) -> (6, -45)
  line L23 (6, 0) -> (20, 0) construction
  line L24 (-6, 0) -> (-20, 0) construction
  line L25 (-6, 6.0184) -> (6, 6.0184)
  line L26 (-6, -6.0184) -> (6, -6.0184)
  line L27 (0, 6.0184) -> (0, -6.0184) construction
  dimension "d93" = 40
  dimension "d94" = 14
  constraint horizontal L16
  constraint vertical L17
  constraint horizontal L18
  constraint vertical L19
  constraint coincident L5 L17.end
  constraint coincident L1 L16.start
  constraint midpoint L16 L20
  constraint coincident L1 L21.start
  constraint coincident L5 L21.end
  constraint perpendicular L5 L21
  constraint coincident L1 L22.start
  constraint coincident L18 L22.end
  constraint perpendicular L18 L22
  constraint midpoint L22 L23.start
  constraint midpoint L17 L23.end
  constraint midpoint L21 L24.start
  constraint midpoint L19 L24.end
  constraint equal L23 L24
  constraint coincident L21 L25.start
  constraint coincident L22 L25.end
  constraint perpendicular L22 L25
  constraint coincident L21 L26.start
  constraint coincident L22 L26.end
  constraint perpendicular L22 L26
  constraint midpoint L25 L27.start
  constraint midpoint L26 L27.end
  constraint midpoint origin L27
  measures "d93" distance of L16.start L16.end
  measures "d94" distance of L24.start L24.end
extrude "Extrude11" add sketch "Sketch9" against normal blind 7 contours L11 L15 L17 L22 | L11 L15 L19 L21 | L21 L22 L25 L26 bodies 1 in component "Bottom"
ref_plane "WorkPlane1" through (-27, 20, 0) normal (1, 0, 0) x (0, 0, -1) in component "Bottom"
sketch "Sketch10" plane through (-20, 0, 0) normal (-1, 0, 0) x (0, 0, 1) in component "Bottom"
  line L0 (-37, 0) -> (37, 0)
  line L1 (37, 0) -> (37, 0.5)
  line L2 (37, 0.5) -> (37, 7)
  line L3 (37, 7) -> (-37, 7)
  line L4 (-37, 7) -> (-37, 0)
  circle A0 centre (22, 5) radius 2
  line L5 (20, 5) -> (20, 7)
  line L6 (24, 5) -> (24, 7)
  line L7 (20, 7) -> (24, 7)
  constraint tangent L3 A0
  constraint coincident A0 L5.start
  constraint coincident L3 L5.end
  constraint perpendicular L3 L5
  constraint coincident A0 L6.start
  constraint coincident L3 L6.end
  constraint perpendicular L3 L6
extrude "Extrude12" cut sketch "Sketch10" against normal blind 40 contours L3 A0 L5 L7 | L3 A0 L6 L7 | A0 bodies 1 in component "Bottom"
sketch "Sketch11" plane through (37, 0, 0) normal (-1, 0, 0) x (0, 0, 1) in component "Bottom"
  line L0 (-33, 40) -> (-33, 0)
  line L1 (-33, 0) -> (33, 0)
  line L2 (33, 0) -> (33, 40)
  line L3 (33, 40) -> (-33, 40)
  circle A0 centre (22, 5) radius 2
extrude "Extrude13" cut sketch "Sketch11" against normal blind 3 contours A0 bodies 1 in component "Bottom"
mirror "Mirror3'" about plane through (0, 0, 0) normal (1, 0, 0) of "Extrude13" in component "Bottom"
sketch "Sketch12" plane through (40, 0, 0) normal (-1, 0, 0) x (0, 0, 1) in component "Bottom"
  circle A0 centre (22, 5) radius 2
  circle A1 centre (22, 5) radius 1.875
  dimension "d104" = 3.75
  constraint concentric A0 A1
  measures "d104" diameter of A1
extrude "Extrude14" add sketch "Sketch12" along normal blind 34 separate body contours A1 makes body 3 in component "Bottom"
mirror "Mirror4" about plane through (0, 0, 0) normal (1, 0, 0) of "Extrude14" makes body 4 in component "Bottom"
ref_plane "WorkPlane1" through (35, 20, 0) normal (-1, 0, 0) x (0, 0, 1) in component "Wheels for tracks"
sketch "Sketch1 (3)" plane through (35, 0, 0) normal (-1, 0, 0) x (0, 0, 1) in component "Wheels for tracks"
  circle A0 centre (22, 5) radius 2.1
  circle A1 centre (22, 5) radius 8
  line L0 (22, 13) -> (22, 12.5) construction
  line L1 (22, 12.5) -> (21.5, 12.5)
  line L2 (21.5, 12.5) -> (21.5, 12.9844)
  line L3 (22, 12.5) -> (22.5, 12.5)
  line L4 (22.5, 12.5) -> (22.5, 12.9844)
  point P0 (22, 5)
  dimension "d110" = 4.2
  dimension "d111" = 16
  constraint coincident P0 A0.centre
  constraint coincident A1 L0.start
  constraint vertical L0
  constraint perpendicular L0 L1
  constraint coincident A1 L2.end
  constraint perpendicular L1 L2
  constraint perpendicular L0 L3
  constraint coincident A1 L4.end
  constraint perpendicular L3 L4
  measures "d110" diameter of A0
  measures "d111" diameter of A1
extrude "Extrude1''" add sketch "Sketch1 (3)" along normal blind 14 separate body makes body 5 in component "Wheels for tracks"
extrude "Extrude2''" cut sketch "Sketch1 (3)" along normal blind 14 contours A1 L1 L2 L3 L4 picked at (22.2223, 12.6661) bodies 5 in component "Wheels for tracks"
pattern_circular "C-Pattern1" count 23 over 360 about axis through (40, 5, 22) along (-1, 0, 0) of "Extrude2''" in component "Wheels for tracks"
mirror "Mirror1" about plane through (0, 0, 0) normal (1, 0, 0) of bodies 5 makes body 6 in component "Wheels for tracks"
sketch "Sketch13" plane through (0, 7, 0) normal (0, 1, 0) x (-1, 0, 0) in component "Bottom"
  line L0 (-6, 20) -> (-20, 20)
  line L1 (-20, 20) -> (-20, -37)
  line L2 (-20, -37) -> (-6, -37)
  line L3 (-6, -37) -> (-6, -6.0184)
  line L4 (-6, -6.0184) -> (6, -6.0184)
  line L5 (6, -6.0184) -> (6, -37)
  line L6 (6, -37) -> (20, -37)
  line L7 (20, -37) -> (20, 20)
  line L8 (20, 20) -> (6, 20)
  line L9 (6, 20) -> (6, 6.0184)
  line L10 (6, 6.0184) -> (-6, 6.0184)
  line L11 (-6, 6.0184) -> (-6, 20)
  line L12 (20, -28.0184) -> (-20, -28.0184)
  line L13 (-20, -28.0184) -> (-20, -16.0184)
  line L14 (-20, -16.0184) -> (20, -16.0184)
  line L15 (20, -16.0184) -> (20, -28.0184)
  dimension "d120" = 12
  dimension "d121" = 10
  constraint horizontal L12
  constraint vertical L13
  constraint horizontal L14
  constraint vertical L15
  constraint coincident L1 L13.end
  constraint coincident L7 L12.start
  measures "d120" distance of L12.start L14.end
  measures "d121" distance of L4 L14
extrude "Extrude15" cut sketch "Sketch13" against normal blind 3 contours L1 L3 L12 L13 L14 | L5 L7 L12 L14 L15 bodies 1 in component "Bottom"
fillet "Fillet1" radius 2.5 4 edges at (-13, 4, -16.0184) (13, 4, -16.0184) (-13, 4, -28.0184) (13, 4, -28.0184) on bodies 1 in component "Bottom"
sketch "Sketch14" plane through (0, 0, 45) normal (0, 0, 1) x (1, 0, 0) in component "Bottom"
  line L0 (-27, 3) -> (2, 3)
  line L1 (-27, 23) -> (-27, 3)
  line L2 (2, 23) -> (-27, 23)
  line L3 (2, 3) -> (2, 23)
  line L4 (-28.5, 1.5) -> (3.5, 1.5)
  line L5 (3.5, 1.5) -> (3.5, 24.5)
  line L6 (3.5, 24.5) -> (-28.5, 24.5)
  line L7 (-28.5, 24.5) -> (-28.5, 1.5)
  dimension "d126" = 1.5
extrude "Extrude16" cut sketch "Sketch14" against normal blind 1 contours L0 L1 L2 L3 | L4 L5 L6 L7 bodies 1 in component "Bottom"
chamfer "Chamfer5'" distance 3 angle 45 4 edges at (-28.5, 1.5, 44.5) (-28.5, 24.5, 44.5) (3.5, 24.5, 44.5) (3.5, 1.5, 44.5) on bodies 1 in component "Bottom"
sketch "Sketch15" plane through (0, 7, 0) normal (0, 1, 0) x (-1, 0, 0) in component "Bottom"
  line L0 (6, 24) -> (20, 24)
  line L1 (20, 24) -> (20, 37)
  line L2 (20, 37) -> (6, 37)
  line L3 (6, 37) -> (6, 24)
  line L4 (-6, 37) -> (37, 37)
  line L5 (37, 37) -> (37, 33)
  line L6 (37, 33) -> (-6, 33)
  line L7 (-6, 33) -> (-6, 37)
  constraint horizontal L4
  constraint vertical L5
  constraint horizontal L6
  constraint vertical L7
extrude "Extrude17" add sketch "Sketch15" against normal blind 7 contours L3 L4 L6 L7 | L1 L4 L5 L6 bodies 1 in component "Bottom"
chamfer "Chamfer6'" distance 4 angle 35 1 edges at (-12.5, 7, 37) measured on face at (-10.3333, 2.6667, 37) on bodies 1 in component "Bottom"
mirror "Mirror2'" about plane through (0, 0, 0) normal (0, 0, 1) of bodies 6 makes body 7 in component "Wheels for tracks"